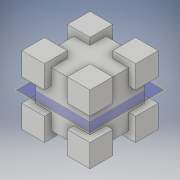
# Autodesk Inventor part: Portal
Saved by Autodesk Inventor 2018 (Build 220112000, 112)
## iProperties
Created: 2020-01-10
Part Number: Portal
Material: Generic
Document SubType Name: Modeling
Designer: AOFUser
Density: 1 g/cm^3
Appearance: Default
Author: AOFUser
Autodesk Inventor part; units mm, degrees
sketch "Sketch1" plane through (0, 0, 0) normal (0, 1, 0) x (-1, 0, 0)
  line L0 (0, 0) -> (-25.4, 0)
  line L1 (-25.4, 0) -> (-25.4, -25.4)
  line L2 (-25.4, -25.4) -> (0, -25.4)
  line L3 (0, -25.4) -> (0, 0)
  dimension "d0" = 25.4
  dimension "d1" = 25.4
  constraints: 8 end point, 2 parallel, 1 horizontal, 1 perpendicular
  measures "d0" distance of L2.end L1.end
  measures "d1" distance of L1.end L0.end
extrude "Extrusion1" add sketch "Sketch1" along normal blind 25.4
sketch "Sketch3" plane through (25.4, 0, 0) normal (1, 0, 0) x (0, 0, -1)
  line L0 (0, 25.4) -> (8.4582, 25.4)
  line L1 (8.4582, 25.4) -> (8.4582, 16.9418)
  line L2 (8.4582, 16.9418) -> (0, 16.9418)
  line L3 (0, 16.9418) -> (0, 25.4)
  line L4 (0, 0) -> (8.4582, 0)
  line L5 (8.4582, 0) -> (8.4582, 8.4582)
  line L6 (8.4582, 8.4582) -> (0, 8.4582)
  line L7 (0, 8.4582) -> (0, 0)
  line L8 (0, 0) -> (25.4, 0) projected
  line L9 (25.4, 0) -> (16.9418, 0)
  line L10 (16.9418, 0) -> (16.9418, 8.4582)
  line L11 (16.9418, 8.4582) -> (25.4, 8.4582)
  line L12 (25.4, 8.4582) -> (25.4, 0)
  line L13 (0, 25.4) -> (25.4, 25.4) projected
  line L14 (25.4, 25.4) -> (16.9418, 25.4)
  line L15 (16.9418, 25.4) -> (16.9418, 16.9418)
  line L16 (16.9418, 16.9418) -> (25.4, 16.9418)
  line L17 (25.4, 16.9418) -> (25.4, 25.4)
  line L18 (8.4582, 25.4) -> (16.9418, 25.4)
  line L19 (16.9418, 25.4) -> (16.9418, 0)
  line L20 (16.9418, 0) -> (8.4582, 0)
  line L21 (8.4582, 0) -> (8.4582, 25.4)
  line L22 (0, 16.9418) -> (25.4, 16.9418)
  line L23 (25.4, 16.9418) -> (25.4, 8.4582)
  line L24 (25.4, 8.4582) -> (0, 8.4582)
  line L25 (0, 8.4582) -> (0, 16.9418)
  dimension "d4" = 8.4582
  dimension "d5" = 8.4582
  dimension "d6" = 8.4582
  dimension "d7" = 8.4582
  dimension "d8" = 8.4582
  dimension "d9" = 8.4582
  dimension "d10" = 8.4582
  dimension "d11" = 8.4582
  constraints: 48 end point, 12 parallel, 6 horizontal, 6 perpendicular
  measures "d4" distance of L1.end L2.end
  measures "d5" distance of L0.end L1.end
  measures "d6" distance of L6.end L5.end
  measures "d7" distance of L5.end L4.end
  measures "d8" distance of L10.end L11.end
  measures "d9" distance of L9.end L10.end
  measures "d10" distance of L16.end L15.end
  measures "d11" distance of L15.end L14.end
extrude "Extrusion2" cut sketch "Sketch3" against normal blind 2.54 contours L13 L15 L22 L1 | L2 L21 L6 L25 | L22 L19 L24 L21 | L24 L10 L8 L5 | L16 L23 L11 L19
sketch "Sketch5" plane through (25.4, 0, -25.4) normal (0, 0, -1) x (-1, 0, 0)
  line L0 (25.4, 0) -> (25.4, 25.4) projected
  line L1 (25.4, 0) -> (16.9418, 0)
  line L2 (16.9418, 0) -> (16.9418, 8.4582)
  line L3 (16.9418, 8.4582) -> (25.4, 8.4582)
  line L4 (25.4, 8.4582) -> (25.4, 0)
  line L5 (0, 0) -> (8.4582, 0)
  line L6 (8.4582, 0) -> (8.4582, 8.4582)
  line L7 (8.4582, 8.4582) -> (0, 8.4582)
  line L8 (0, 8.4582) -> (0, 0)
  line L9 (2.54, 25.4) -> (0, 25.4) projected
  line L10 (0, 25.4) -> (8.4582, 25.4)
  line L11 (8.4582, 25.4) -> (8.4582, 16.9418)
  line L12 (8.4582, 16.9418) -> (0, 16.9418)
  line L13 (0, 16.9418) -> (0, 25.4)
  line L14 (0, 25.4) -> (25.4, 25.4) projected
  line L15 (25.4, 25.4) -> (16.9418, 25.4)
  line L16 (16.9418, 25.4) -> (16.9418, 16.9418)
  line L17 (16.9418, 16.9418) -> (25.4, 16.9418)
  line L18 (25.4, 16.9418) -> (25.4, 25.4)
  line L19 (0, 8.4582) -> (2.54, 8.4582) projected
  line L20 (0, 8.4582) -> (25.4, 8.4582)
  line L21 (25.4, 8.4582) -> (25.4, 16.9418)
  line L22 (25.4, 16.9418) -> (0, 16.9418)
  line L23 (0, 16.9418) -> (0, 8.4582)
  line L24 (8.4582, 25.4) -> (16.9418, 25.4)
  line L25 (16.9418, 25.4) -> (16.9418, 0)
  line L26 (16.9418, 0) -> (8.4582, 0)
  line L27 (8.4582, 0) -> (8.4582, 25.4)
  dimension "d14" = 8.4582
  dimension "d15" = 8.4582
  dimension "d16" = 8.4582
  dimension "d17" = 8.4582
  dimension "d18" = 8.4582
  dimension "d19" = 8.4582
  dimension "d20" = 8.4582
  dimension "d21" = 8.4582
  constraints: 48 end point, 12 parallel, 6 horizontal, 6 perpendicular
  measures "d14" distance of L2.end L3.end
  measures "d15" distance of L1.end L2.end
  measures "d16" distance of L7.end L6.end
  measures "d17" distance of L6.end L5.end
  measures "d18" distance of L11.end L12.end
  measures "d19" distance of L10.end L11.end
  measures "d20" distance of L17.end L16.end
  measures "d21" distance of L16.end L15.end
extrude "Extrusion3" cut sketch "Sketch5" against normal blind 2.54 contours L3 L25 L17 L0 | L26 L6 L20 L2 | L20 L27 L22 L25 | L22 L11 L14 L16 | L7 L23 L12 L27
sketch "Sketch7" plane through (0, 0, 0) normal (0, -1, 0) x (1, 0, 0)
  line L0 (25.4, -16.9418) -> (25.4, -25.4) projected
  line L1 (25.4, -25.4) -> (16.9418, -25.4)
  line L2 (16.9418, -25.4) -> (16.9418, -16.9418)
  line L3 (16.9418, -16.9418) -> (25.4, -16.9418)
  line L4 (25.4, -16.9418) -> (25.4, -25.4)
  line L5 (8.4582, -25.4) -> (0, -25.4) projected
  line L6 (0, -25.4) -> (8.4582, -25.4)
  line L7 (8.4582, -25.4) -> (8.4582, -16.9418)
  line L8 (8.4582, -16.9418) -> (0, -16.9418)
  line L9 (0, -16.9418) -> (0, -25.4)
  line L10 (25.4, -8.4582) -> (25.4, 0) projected
  line L11 (25.4, 0) -> (16.9418, 0)
  line L12 (16.9418, 0) -> (16.9418, -8.4582)
  line L13 (16.9418, -8.4582) -> (25.4, -8.4582)
  line L14 (25.4, -8.4582) -> (25.4, 0)
  line L15 (0, 0) -> (25.4, 0) projected
  line L16 (0, 0) -> (8.4582, 0)
  line L17 (8.4582, 0) -> (8.4582, -8.4582)
  line L18 (8.4582, -8.4582) -> (0, -8.4582)
  line L19 (0, -8.4582) -> (0, 0)
  line L20 (16.9418, -25.4) -> (8.4582, -25.4)
  line L21 (8.4582, -25.4) -> (8.4582, 0)
  line L22 (8.4582, 0) -> (16.9418, 0)
  line L23 (16.9418, 0) -> (16.9418, -25.4)
  line L24 (0, -16.9418) -> (25.4, -16.9418)
  line L25 (25.4, -16.9418) -> (25.4, -8.4582)
  line L26 (25.4, -8.4582) -> (0, -8.4582)
  line L27 (0, -8.4582) -> (0, -16.9418)
  dimension "d32" = 8.4582
  dimension "d33" = 8.4582
  dimension "d34" = 8.4582
  dimension "d35" = 8.4582
  dimension "d36" = 8.4582
  dimension "d37" = 8.4582
  dimension "d38" = 8.4582
  dimension "d39" = 8.4582
  constraints: 48 end point, 12 parallel, 6 horizontal, 6 perpendicular
  measures "d32" distance of L2.end L3.end
  measures "d33" distance of L1.end L2.end
  measures "d34" distance of L8.end L7.end
  measures "d35" distance of L7.end L6.end
  measures "d36" distance of L13.end L12.end
  measures "d37" distance of L12.end L11.end
  measures "d38" distance of L17.end L18.end
  measures "d39" distance of L16.end L17.end
extrude "Extrusion4" cut sketch "Sketch7" against normal blind 2.54 contours L3 L23 L13 L25 | L24 L21 L26 L23 | L2 L20 L7 L24 | L26 L17 L15 L12 | L8 L27 L18 L21
ref_plane "Work Plane1" through (12.7, 0, 0) normal (1, 0, 0) x (0, 1, 0)
ref_plane "Work Plane2" through (0, 12.7, 0) normal (0, 1, 0) x (-1, 0, 0)
ref_plane "Work Plane3" through (0, 0, -12.7) normal (0, 0, 1) x (1, 0, 0)
mirror "Mirror1" about plane through (12.7, 0, 0) normal (1, 0, 0) of "Extrusion2"
mirror "Mirror2" about plane through (0, 0, -12.7) normal (0, 0, 1) of "Extrusion3"
mirror "Mirror3" about plane through (0, 12.7, 0) normal (0, 1, 0) of "Extrusion4"
ref_plane "Work Plane4" through (0, 12.7, 0) normal (0, 1, 0) x (-1, 0, 0)
body "Solid1"
